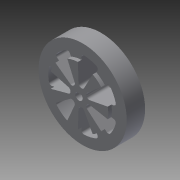
# Autodesk Inventor part: Wheel Printable
Saved by Autodesk Inventor 2013 SP2 (Build 170200200, 200)
## iProperties
Created: 2014-04-23
Part Number: Wheel Printable
Material: Generic
Document SubType Name: Modeling
Designer: Kevin
Density: 1 g/cm^3
Author: Kevin
Autodesk Inventor part; units mm, degrees
ref_plane "YZ Plane" through (0, 0, 0) normal (1, 0, 0) x (0, 1, 0)
ref_plane "XZ Plane" through (0, 0, 0) normal (0, 1, 0) x (-1, 0, 0)
ref_plane "XY Plane" through (0, 0, 0) normal (0, 0, 1) x (1, 0, 0)
sketch "Sketch1" plane through (0, 0, 0) normal (0, 0, 1) x (1, 0, 0)
  circle A0 centre (0, 0) radius 18
  dimension "d0" = 36
  constraints: 1 centre point, 1 coincident
  measures "d0" diameter of A0
extrude "Extrusion1" add sketch "Sketch1" against normal blind 9
sketch "Sketch2" plane through (0, 0, 0) normal (0, 0, 1) x (1, 0, 0)
  circle A0 centre (0, 0) radius 18 projected
  circle A1 centre (0, 0) radius 16
  circle A2 centre (0, 0) radius 11.95
  dimension "d3" = 32
  dimension "d4" = 23.9
  constraints: 2 centre point, 2 coincident
  measures "d3" diameter of A1
  measures "d4" diameter of A2
extrude "Extrusion2" cut sketch "Sketch2" against normal blind 1.5 contours A0 | A1
sketch "Sketch3" plane through (0, 0, 0) normal (0, 0, 1) x (1, 0, 0)
  circle A0 centre (0, 0) radius 11.95 projected
  arc A1 (-1.118, 1) -> (1.118, 1) centre (0, 0) ccw
  line L0 (0, 0) -> (0, 1)
  line L1 (0, 1) -> (-1.118, 1)
  line L2 (0, 1) -> (1.118, 1)
  arc A2 (1.118, 1) -> (-1.118, 1) centre (0, 0) ccw
  dimension "d7" = 3
  dimension "d8" = 1
  constraints: 6 end point, 4 point on circle, 2 centre point, 1 coincident, 1 collinear, 1 perpendicular, 1 vertical
  measures "d7" diameter of A1
  measures "d8" distance of L0.start L0.end
extrude "Extrusion3" cut sketch "Sketch3" against normal blind 8 contours L1 L2 A1
sketch "Sketch4" plane through (0, 0, -9) normal (0, 0, -1) x (-1, 0, 0)
  circle A0 centre (0, 0) radius 18 projected
  circle A1 centre (0, 0) radius 1.5
  arc A2 (3.4975, -0.1319) -> (3.4975, 0.1319) centre (0, 0) ccw
  arc A3 (13.7616, -2.5725) -> (13.7616, 2.5725) centre (0, 0) ccw
  line L0 (0, 0) -> (16, 0) construction
  line L1 (0, 0) -> (16, 0) construction
  line L2 (4.238, 1.1356) -> (12.5198, 3.3547)
  line L3 (4.238, -1.1356) -> (12.5198, -3.3547)
  arc A4 (4.238, 1.1356) -> (3.4975, 0.1319) centre (4.4968, 0.1696) ccw
  arc A5 (13.7616, 2.5725) -> (12.5198, 3.3547) centre (12.7786, 2.3888) ccw
  arc A6 (12.5198, -3.3547) -> (13.7616, -2.5725) centre (12.7786, -2.3888) ccw
  arc A7 (3.4975, -0.1319) -> (4.238, -1.1356) centre (4.4968, -0.1696) ccw
  arc A8 (2.2838, 2.6522) -> (2.0775, 2.8167) centre (0, 0) ccw
  arc A9 (10.5915, 9.1553) -> (6.569, 12.3632) centre (0, 0) ccw
  line L4 (1.7545, 4.0214) -> (5.1832, 11.88)
  line L5 (3.5302, 2.6054) -> (10.4288, 7.6968)
  arc A10 (1.7545, 4.0214) -> (2.0775, 2.8167) centre (2.6711, 3.6215) ccw
  arc A11 (6.569, 12.3632) -> (5.1832, 11.88) centre (6.0998, 11.4801) ccw
  arc A12 (10.4288, 7.6968) -> (10.5915, 9.1553) centre (9.835, 8.5014) ccw
  arc A13 (2.2838, 2.6522) -> (3.5302, 2.6054) centre (2.9363, 3.41) ccw
  arc A14 (-0.6496, 3.4392) -> (-0.9069, 3.3805) centre (0, 0) ccw
  arc A15 (-0.5542, 13.989) -> (-5.5703, 12.8442) centre (0, 0) ccw
  line L6 (-2.0501, 3.879) -> (-6.0565, 11.4594)
  line L7 (0.1641, 4.3844) -> (0.4846, 12.9524)
  arc A16 (-2.0501, 3.879) -> (-0.9069, 3.3805) centre (-1.166, 4.3463) ccw
  arc A17 (-5.5703, 12.8442) -> (-6.0565, 11.4594) centre (-5.1724, 11.9267) ccw
  arc A18 (0.4846, 12.9524) -> (-0.5542, 13.989) centre (-0.5147, 12.9898) ccw
  arc A19 (-0.6496, 3.4392) -> (0.1641, 4.3844) centre (-0.8352, 4.4218) ccw
  arc A20 (-3.0939, 1.6364) -> (-3.2084, 1.3986) centre (0, 0) ccw
  arc A21 (-11.2826, 8.2887) -> (-13.515, 3.6532) centre (0, 0) ccw
  line L8 (-4.311, 0.8157) -> (-12.7355, 2.4097)
  line L9 (-3.3256, 2.8619) -> (-9.8244, 8.4546)
  arc A22 (-4.311, 0.8157) -> (-3.2084, 1.3986) centre (-4.1251, 1.7983) ccw
  arc A23 (-13.515, 3.6532) -> (-12.7355, 2.4097) centre (-12.5496, 3.3923) ccw
  arc A24 (-9.8244, 8.4546) -> (-11.2826, 8.2887) centre (-10.4767, 7.6966) ccw
  arc A25 (-3.0939, 1.6364) -> (-3.3256, 2.8619) centre (-3.9779, 2.1039) ccw
  arc A26 (-3.2084, -1.3986) -> (-3.0939, -1.6364) centre (0, 0) ccw
  arc A27 (-13.515, -3.6532) -> (-11.2826, -8.2887) centre (0, 0) ccw
  line L10 (-3.3256, -2.8619) -> (-9.8244, -8.4546)
  line L11 (-4.311, -0.8157) -> (-12.7355, -2.4097)
  arc A28 (-3.3256, -2.8619) -> (-3.0939, -1.6364) centre (-3.9779, -2.1039) ccw
  arc A29 (-11.2826, -8.2887) -> (-9.8244, -8.4546) centre (-10.4767, -7.6966) ccw
  arc A30 (-12.7355, -2.4097) -> (-13.515, -3.6532) centre (-12.5496, -3.3923) ccw
  arc A31 (-3.2084, -1.3986) -> (-4.311, -0.8157) centre (-4.1251, -1.7983) ccw
  arc A32 (-0.9069, -3.3805) -> (-0.6496, -3.4392) centre (0, 0) ccw
  arc A33 (-5.5703, -12.8442) -> (-0.5542, -13.989) centre (0, 0) ccw
  line L12 (0.1641, -4.3844) -> (0.4846, -12.9524)
  line L13 (-2.0501, -3.879) -> (-6.0565, -11.4594)
  arc A34 (0.1641, -4.3844) -> (-0.6496, -3.4392) centre (-0.8352, -4.4218) ccw
  arc A35 (-0.5542, -13.989) -> (0.4846, -12.9524) centre (-0.5147, -12.9898) ccw
  arc A36 (-6.0565, -11.4594) -> (-5.5703, -12.8442) centre (-5.1724, -11.9267) ccw
  arc A37 (-0.9069, -3.3805) -> (-2.0501, -3.879) centre (-1.166, -4.3463) ccw
  arc A38 (2.0775, -2.8167) -> (2.2838, -2.6522) centre (0, 0) ccw
  arc A39 (6.569, -12.3632) -> (10.5915, -9.1553) centre (0, 0) ccw
  line L14 (3.5302, -2.6054) -> (10.4288, -7.6968)
  line L15 (1.7545, -4.0214) -> (5.1832, -11.88)
  arc A40 (3.5302, -2.6054) -> (2.2838, -2.6522) centre (2.9363, -3.41) ccw
  arc A41 (10.5915, -9.1553) -> (10.4288, -7.6968) centre (9.835, -8.5014) ccw
  arc A42 (5.1832, -11.88) -> (6.569, -12.3632) centre (6.0998, -11.4801) ccw
  arc A43 (2.0775, -2.8167) -> (1.7545, -4.0214) centre (2.6711, -3.6215) ccw
  dimension "d11" = 3
  dimension "d13" = 28
  dimension "d16" = 1
  dimension "d19" = 360
  constraints: 84 point on circle, 43 centre point, 32 end point, 9 coincident, 8 tangent, 3 equal radius, 2 horizontal, 155 other
  measures "d11" diameter of A1
  measures "d13" diameter of A3
  measures "d16" radius of A4
extrude "Extrusion4" cut sketch "Sketch4" against normal blind 12 contours A2 A4 L2 A5 A3 A6 L3 A7 | A8 A10 L4 A11 A9 A12 L5 A13 | A14 A16 L6 A17 A15 A18 L7 A19 | A20 A22 L8 A23 A21 A24 L9 A25 | A26 A28 L10 A29 A27 A30 L11 A31 | A32 A34 L12 A35 A33 A36 L13 A37 | A38 A40 L14 A41 A39 A42 L15 A43
fillet "Fillet1" radius 0.5 56 edges at (-2.8988, 2.4107, -9) (-2.1822, 2.7364, -9) (-1.7052, 3.3625, -9) (-3.4689, 7.9507, -9) (-5.7705, 12.4244, -9) (-8.7289, 10.9456, -9) (-10.8288, 8.3905, -9) (-6.9795, 5.1511, -9) (0.0774, 3.7694, -9) (0.7788, 3.4122, -9) (1.5658, 3.4297, -9) (4.0533, 7.6692, -9) (6.1159, 12.258, -9) (3.1153, 13.649, -9) (-0.1917, 13.6977, -9) (-0.3243, 8.6684, -9) (2.9953, 2.2897, -9) (3.1534, 1.5186, -9) (3.6577, 0.9142, -9) (8.5233, 1.6127, -9) (13.3969, 2.8612, -9) (12.6136, 6.0744, -9) (10.5898, 8.6902, -9) (6.575, 5.6583, -9) (3.6577, -0.9142, -9) (3.1534, -1.5186, -9) (2.9953, -2.2897, -9) (6.575, -5.6583, -9) (10.5898, -8.6902, -9) (12.6136, -6.0744, -9) (13.3969, -2.8612, -9) (8.5233, -1.6127, -9) (-0.1917, -13.6977, -9) (3.1153, -13.649, -9) (6.1159, -12.258, -9) (4.0533, -7.6692, -9) (1.5658, -3.4297, -9) (0.7788, -3.4122, -9) (0.0774, -3.7694, -9) (-0.3243, -8.6684, -9) (-10.8288, -8.3905, -9) (-8.7289, -10.9456, -9) (-5.7705, -12.4244, -9) (-3.4689, -7.9507, -9) (-1.7052, -3.3625, -9) (-2.1822, -2.7364, -9) (-2.8988, -2.4107, -9) (-6.9795, -5.1511, -9) (-3.6921, -0.7633, -9) (-3.5, 0, -9) (-3.6921, 0.7633, -9) (-8.3789, 2.2451, -9) (-13.3116, 3.2349, -9) (-14, 0, -9) (-13.3116, -3.2349, -9) (-8.3789, -2.2451, -9)
body "Solid1"
